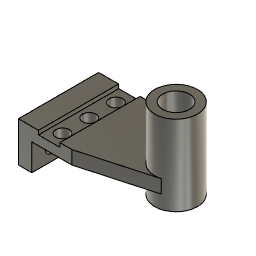
Part 15 (Autodesk Fusion 360 design; units mm, degrees)
Autodesk Fusion 360 part; units mm, degrees
note: some values were not read from the file. Chosen so that the rebuilt part matches the saved one: a direction.
sketch "Sketch2" plane through (0, 0, 0) normal (0, 0, 1) x (1, 0, 0)
  circle A0 centre (0, 0) radius 16
  line L0 (4.2989, 15.4117) -> (-48, 30)
  line L1 (-48, 30) -> (-88, 30)
  line L2 (-88, 30) -> (-88, -30)
  line L3 (-88, -30) -> (-48, -30)
  line L4 (-48, -30) -> (4.2989, -15.4117)
  line L5 (0, 0) -> (-88, 0) construction
  circle A1 centre (0, 0) radius 10
  dimension "d12" = 32
  dimension "d13" = 88
  dimension "d14" = 60
  dimension "d15" = 40
  dimension "d16" = 30
  dimension "d17" = 20
  constraint coincident A0.centre L5.start
  constraint coincident A0 L0.start
  constraint horizontal L1
  constraint perpendicular L1 L2
  constraint perpendicular L2 L3
  constraint coincident A0 L4.end
  constraint tangent A0 L4
  constraint tangent A0 L0
  constraint perpendicular L2 L5
  constraint coincident L2 L5.end
  constraint equal L1 L3
  constraint concentric A0 A1
  measures "d12" diameter of A0
  measures "d13" distance of A0.centre L5.end
  measures "d14" distance of L1.end L2.end
  measures "d15" distance of L0.end L1.end
  measures "d16" distance of L1 L5
  measures "d17" diameter of A1
extrude "Extrude2" add sketch "Sketch2" against normal blind 10 contours A0 L0 L1 L2 L3 L4
extrude "Extrude3" add sketch "Sketch2" along normal blind 40 and the other way blind 20 contours A0
sketch "Sketch3" plane through (0, 0, 0) normal (0, 0, 1) x (-1, 0, 0)
  line L0 (-4.2989, -15.4117) -> (48, -30)
  line L1 (48, -30) -> (88, -30)
  line L2 (88, -30) -> (88, 30)
  line L3 (88, 30) -> (48, 30)
  line L4 (48, 30) -> (-4.2989, 15.4117)
  arc A0 (-4.2989, -15.4117) -> (-4.2989, 15.4117) centre (0, 0) ccw
  line L5 (73, -30) -> (57, -30)
  line L6 (57, -30) -> (57, 30)
  line L7 (57, 30) -> (73, 30)
  line L8 (73, 30) -> (73, -30)
  circle A1 centre (65, 20) radius 5
  dimension "d24" = 15
  dimension "d25" = 16
  dimension "d26" = 10
  dimension "d27" = 10
  dimension "d28" = 8
  constraint horizontal L5
  constraint vertical L6
  constraint horizontal L7
  constraint vertical L8
  constraint coincident L3 L6.end
  constraint coincident L1 L5.start
  measures "d24" distance of L2 L8
  measures "d25" distance of L6 L8
  measures "d26" diameter of A1
  measures "d27" distance of L7 A1.centre
  measures "d28" distance of L8 A1.centre
extrude "Extrude4" cut sketch "Sketch3" against normal blind 3 contours L1 L3 L5 L6 L7 L8
extrude "Extrude5" cut 1 faces at (-64.762, -19.9266, 0) along direction (0, 0, -1) through all
sketch "Sketch4" plane through (0, 0, -10) normal (0, 0, -1) x (1, 0, 0)
  circle A0 centre (-65, 20) radius 5
  line L0 (-48, -30) -> (4.2989, -15.4117)
  arc A1 (4.2989, 15.4117) -> (4.2989, -15.4117) centre (0, 0) ccw
  line L1 (4.2989, 15.4117) -> (-48, 30)
  line L2 (-48, 30) -> (-88, 30)
  line L3 (-88, 30) -> (-88, -30)
  line L4 (-88, -30) -> (-48, -30)
  line L5 (-88, 30) -> (-78, 30)
  line L6 (-78, 30) -> (-78, -30)
  line L7 (-78, -30) -> (-88, -30)
  line L8 (-88, -30) -> (-88, 30)
  dimension "d35" = 10
  constraint horizontal L5
  constraint vertical L6
  constraint horizontal L7
  constraint vertical L8
  constraint coincident L4 L6.end
  constraint coincident L2.end L3.start
  measures "d35" distance of L6 L8
extrude "Extrude6" add sketch "Sketch4" along normal blind 20 contours L2 L3 L4 L5 L6 L7 L8
pattern_linear "R-Pattern1" count 3 spacing 20 along (0, 1, 0) of "Extrude5"
sketch "Sketch5" plane through (-88, 0, 0) normal (-1, 0, 0) x (0, -1, 0)
  line L0 (30, 0) -> (-30, 0)
  line L1 (-30, 0) -> (-30, -30)
  line L2 (-30, -30) -> (30, -30)
  line L3 (30, -30) -> (30, 0)
  circle A0 centre (-15, -20) radius 5
  dimension "d42" = 10
  dimension "d43" = 15
  dimension "d44" = 10
  measures "d42" diameter of A0
  measures "d43" distance of L1 A0.centre
  measures "d44" distance of L2 A0.centre
extrude "Extrude7" cut sketch "Sketch5" against normal blind 10 contours A0
pattern_linear "R-Pattern2" count 2 spacing 30 along (0, -1, 0) of "Extrude7"
